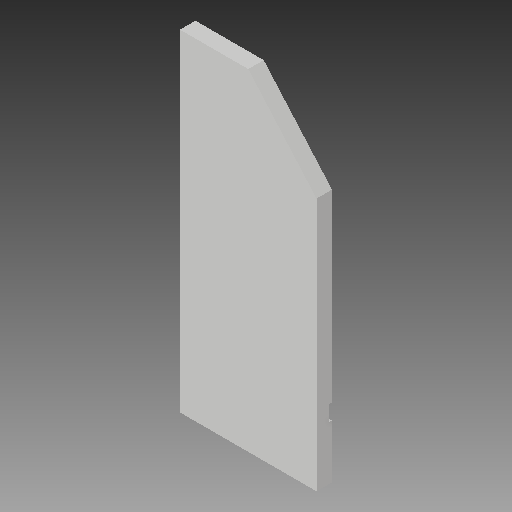
# Autodesk Inventor part: LATERAL_BLOCOS_BASE
Saved by Autodesk Inventor 2018 (Build 220112000, 112)
## iProperties
Created: 2018-10-09
Part Number: LATERAL_BLOCOS_BASE
Material: Genérico
Document SubType Name: Modeling
Designer: Georgines
Density: 1 g/cm^3
Appearance: Padrão
Author: Georgines
Autodesk Inventor part; units mm, degrees
ref_plane "YZ Plane" through (0, 0, 0) normal (1, 0, 0) x (0, 1, 0)
ref_plane "XZ Plane" through (0, 0, 0) normal (0, 1, 0) x (-1, 0, 0)
ref_plane "XY Plane" through (0, 0, 0) normal (0, 0, 1) x (1, 0, 0)
sketch "Esboço1" plane through (0, 0, 0) normal (0, 0, 1) x (1, 0, 0)
  line L0 (0, 306.9957) -> (70, 306.9957)
  line L1 (140, 226.9957) -> (140, -33.0043)
  line L2 (140, -33.0043) -> (0, -33.0043)
  line L3 (0, -33.0043) -> (0, 306.9957)
  line L4 (70, 306.9957) -> (140, 226.9957)
  dimension "d0" = 140
  dimension "d1" = 340
  dimension "d2" = 70
  dimension "d3" = 260
  constraints: 10 end point, 2 parallel, 1 horizontal, 1 perpendicular
  measures "d0" distance of L1.end L2.end
  measures "d1" distance of L2.end L0.start
  measures "d2" distance of L0.start L0.end
  measures "d3" distance of L1.start L1.end
extrude "Extrusão1" add sketch "Esboço1" along normal blind 15.88
sketch "Esboço3" plane through (0, 0, 0) normal (0, 0, -1) x (-1, 0, 0)
  line L0 (0, 21.9457) -> (-140, 21.9457)
  line L1 (0, 21.9457) -> (0, 37.9257)
  line L2 (-140, 37.9257) -> (0, 37.9257)
  line L3 (-140, 21.9457) -> (-140, 37.9257)
  line L4 (-140, -33.0043) -> (-140, 226.9957) construction
  line L5 (-140, 29.9357) -> (0, 29.9357) construction
  point P0 (0, 0)
  dimension "d11" = 15.98
  constraints: 10 end point, 1 horizontal, 1 midpoint, 1 point on line
  measures "d11" distance of L0.start L1.end
extrude "Extrusão3" cut sketch "Esboço3" against normal blind 3
